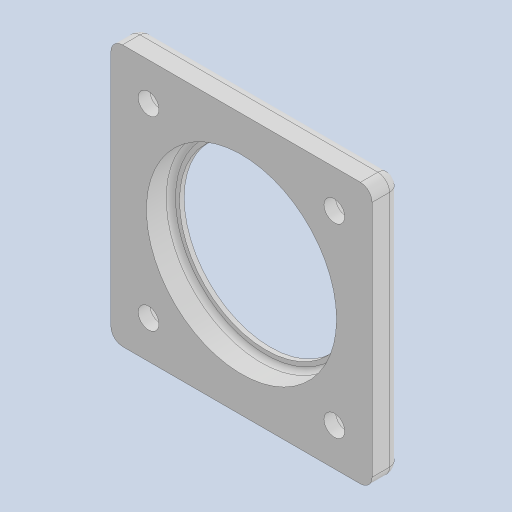
# Autodesk Inventor part: cage_inside_01
Saved by Autodesk Inventor 2024.4 (Build 284460000, 460)
## iProperties
Created: 2026-03-25
Part Number: cage_inside_01
Material: Generic
Document SubType Name: Modeling
Designer: tooles01
Density: 1 g/cm^3
Appearance: Default
Author: tooles01
Autodesk Inventor part; units mm, degrees
ref_plane "YZ Plane" through (0, 0, 0) normal (1, 0, 0) x (0, 1, 0)
ref_plane "XZ Plane" through (0, 0, 0) normal (0, 1, 0) x (-1, 0, 0)
ref_plane "XY Plane" through (0, 0, 0) normal (0, 0, 1) x (1, 0, 0)
sketch "Sketch1: base" plane through (0, 0, 0) normal (0, 0, 1) x (1, 0, 0)
  line L0 (-22.9459, 27.4044) -> (22.0541, 27.4044)
  line L1 (22.0541, 27.4044) -> (22.0541, -17.5956)
  line L2 (22.0541, -17.5956) -> (-22.9459, -17.5956)
  line L3 (-22.9459, -17.5956) -> (-22.9459, 27.4044)
  circle A0 centre (-0.4459, 4.9044) radius 16.375
  line L4 (-16.4459, 20.9044) -> (15.5541, 20.9044) construction
  line L5 (15.5541, 20.9044) -> (15.5541, -11.0956) construction
  line L6 (15.5541, -11.0956) -> (-16.4459, -11.0956) construction
  line L7 (-16.4459, -11.0956) -> (-16.4459, 20.9044) construction
  circle A1 centre (-0.4459, 4.9044) radius 14.875
  circle A2 centre (15.5541, 20.9044) radius 1.8 construction
  circle A3 centre (15.5541, 20.9044) radius 3.25 construction
  point P0 (0, 0)
  point P1 (22.0541, 4.9044)
  point P2 (-0.4459, 27.4044)
  point P3 (-0.4459, 20.9044)
  point P4 (-16.4459, 4.9044)
  dimension "d0" = 32.75
  dimension "d1" = 45
  dimension "d4" = 32
  dimension "d16" = 1.5
  dimension "d19" = 6.5
  dimension "d20" = 3.6
  dimension "d21" = 6.5
  constraints: 16 end point, 8 perpendicular, 7 coincident, 4 centre point, 4 midpoint, 2 horizontal, 2 horizontal alignment, 2 vertical alignment, 1 other
  measures "d0" diameter of A0
  measures "d1" distance of L0.start L0.end
  measures "d4" distance of L4.start L4.end
  measures "d16" radial gap between concentric circles of A1 A0
  measures "d19" distance between parallel lines of L1 L5
  measures "d20" diameter of A2
  measures "d21" diameter of A3
extrude "Ex1: base" add sketch "Sketch1: base" along normal blind 5 contours L0 L1 L2 L3
hole "Hole1: M3 screws" at (-16.4459, 20.9044, 0) at (15.5541, 20.9044, 0) at (-16.4459, -11.0956, 0) at (15.5541, -11.0956, 0) direction (0, 0, 1) diameter 3.6 end through all counterbore diameter 6.5 counterbore depth 3 clearance for "Socket Head Cap Screw" size "M3" standard "Ansi Metric M Profile"
fillet "Fillet1" radius 2 8 edges at (-0.4459, 27.4044, 0) (22.0541, 4.9044, 0) (22.0541, 27.4044, 2.5) (-22.9459, 4.9044, 0) (-0.4459, -17.5956, 0) (22.0541, -17.5956, 2.5) (-22.9459, -17.5956, 2.5) (-22.9459, 27.4044, 2.5)
extrude "Ex2: stopper" add sketch "Sketch1: base" along normal blind 0.8 contours A0
fillet "Fillet2 (for printing)" radius 0.8 1 edges at (-16.8209, 4.9044, 0.8)
body "Solid1"
